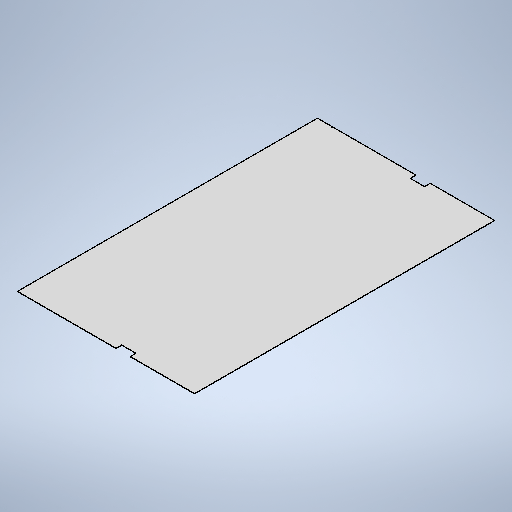
# Autodesk Inventor part: GnG frame 1.1 floor sheet 2
Saved by Autodesk Inventor 2025.3 (Build 293356000, 356)
## iProperties
Created: 2025-10-28
Part Number: GnG frame 1.1 floor sheet 2
Material: Stainless Steel
Document SubType Name: Sheet Metal
Designer: admin
Mass: 280.619 g
Surface Area: 364.406 cm^2
Volume: 35.0774 cm^3
Density: 8 g/cm^3
Sheet Metal Rule: AISI304 3mm Die 32
Sheet Metal Width: 1240,000 mm
Sheet Metal Length: 2100,000 mm
Sheet Metal Area: 2604000,000 mm^2
Appearance: Default
Stock Number: 1.2
Flat Pattern Width: 124 cm
Flat Pattern Length: 210 cm
Flat Pattern Area: 26040 cm^2
Author: admin
Autodesk Inventor part; units mm, degrees
ref_plane "YZ Plane" through (0, 0, 0) normal (1, 0, 0) x (0, 1, 0)
ref_plane "XZ Plane" through (0, 0, 0) normal (0, 1, 0) x (-1, 0, 0)
ref_plane "XY Plane" through (0, 0, 0) normal (0, 0, 1) x (1, 0, 0)
sketch "Sketch1" plane through (0, 0, 0) normal (0, 0, 1) x (1, 0, 0)
  line L0 (0, 0) -> (-1240, 0)
  line L1 (-1240, 0) -> (-1240, -2100)
  line L2 (-1240, -2100) -> (0, -2100)
  line L3 (0, -2100) -> (0, 0)
  line L4 (0, 0) -> (-40, 0)
  line L5 (-40, 0) -> (-40, -40)
  line L6 (-40, -40) -> (0, -40)
  line L7 (0, -40) -> (0, 0)
  line L8 (0, -2100) -> (-40, -2100)
  line L9 (-40, -2100) -> (-40, -2060)
  line L10 (-40, -2060) -> (0, -2060)
  line L11 (0, -2060) -> (0, -2100)
  line L12 (-1240, 0) -> (-1200, 0)
  line L13 (-1200, 0) -> (-1200, -40)
  line L14 (-1200, -40) -> (-1240, -40)
  line L15 (-1240, -40) -> (-1240, 0)
  line L16 (-1240, -2100) -> (-1200, -2100)
  line L17 (-1200, -2100) -> (-1200, -2060)
  line L18 (-1200, -2060) -> (-1240, -2060)
  line L19 (-1240, -2060) -> (-1240, -2100)
  line L20 (-550, -2100) -> (-450, -2100)
  line L21 (-450, -2100) -> (-450, -2060)
  line L22 (-450, -2060) -> (-550, -2060)
  line L23 (-550, -2060) -> (-550, -2100)
  line L24 (-550, 0) -> (-450, 0)
  line L25 (-450, 0) -> (-450, -40)
  line L26 (-450, -40) -> (-550, -40)
  line L27 (-550, -40) -> (-550, 0)
  point P0 (0, -40)
  point P1 (-40, 0)
  point P2 (-40, -2100)
  point P3 (0, -2060)
  point P4 (-450, -2100)
  point P5 (-450, 0)
  dimension "d22" = 1240
  dimension "d23" = 2100
  dimension "d24" = 40
  dimension "d25" = 40
  dimension "d28" = 100
  dimension "d29" = 410
  measures "d22" distance of L2.end L1.end
  measures "d23" distance of L1.end L0.end
  measures "d24" distance of L6.end L5.end
  measures "d25" distance of L5.end L4.end
  measures "d28" distance of L25.end L26.end
  measures "d29" distance between parallel lines of L5 L25
extrude "Plate1" add sketch "Sketch1" along normal blind 3 contours L3 L6 L5 L0 | L5 L6 L3 L10 L9 L2 L21 L22 L23 L17 L18 L1 L14 L13 L0 L27 L26 L25 | L3 L2 L9 L10 | L13 L14 L1 L0 | L18 L17 L2 L1
sketch "Sketch6" plane through (0, 0, 3) normal (0, 0, 1) x (1, 0, 0)
  line L0 (0, 0) -> (0, -2100) projected
  line L1 (-450, 0) -> (0, 0) projected
  line L2 (-450, -40) -> (-450, 0) projected
  line L3 (-550, -40) -> (-450, -40) projected
  line L4 (-550, 0) -> (-550, -40) projected
  line L5 (-1240, 0) -> (-550, 0) projected
  line L6 (-1240, -2100) -> (-1240, 0) projected
  line L7 (-550, -2100) -> (-1240, -2100) projected
  line L8 (-550, -2060) -> (-550, -2100) projected
  line L9 (-450, -2060) -> (-550, -2060) projected
  line L10 (-450, -2100) -> (-450, -2060) projected
  line L11 (0, -2100) -> (-450, -2100) projected
  line L12 (-1135, 0) -> (-1133, 0)
  line L13 (-1133, 0) -> (-1133, -5)
  line L14 (-1133, -5) -> (-1135, -5)
  line L15 (-1135, -5) -> (-1135, 0)
  line L16 (-1127, 0) -> (-1125, 0)
  line L17 (-1125, 0) -> (-1125, -5)
  line L18 (-1125, -5) -> (-1127, -5)
  line L19 (-1127, -5) -> (-1127, 0)
  line L20 (-1131, 0) -> (-1129, 0)
  line L21 (-1129, 0) -> (-1129, -5)
  line L22 (-1129, -5) -> (-1131, -5)
  line L23 (-1131, -5) -> (-1131, 0)
  line L24 (-1133, -2.5) -> (-1131, -2.5)
  line L25 (-1123, 0) -> (-1120, 0)
  line L26 (-1129, -2.5) -> (-1127, -2.5)
  line L27 (-1123, 0) -> (-1121.9884, -4.6072)
  arc A0 (-1121.9884, -4.6072) -> (-1121.0116, -4.6072) centre (-1121.5, -4.5) ccw
  line L28 (-1121.0116, -4.6072) -> (-1120, 0)
  line L29 (-1125, 0) -> (-1123, 0)
  line L30 (-1112, -5) -> (-1114, -5)
  line L31 (-1112, -2.5) -> (-1110, -2.5)
  line L32 (-1116, -5) -> (-1118, -5)
  line L33 (-1116, -2.5) -> (-1114, -2.5)
  line L34 (-1114, 0) -> (-1112, 0)
  line L35 (-1114, -5) -> (-1114, 0)
  line L36 (-1118, 0) -> (-1116, 0)
  line L37 (-1118, -5) -> (-1118, 0)
  line L38 (-1116, 0) -> (-1116, -5)
  line L39 (-1112, 0) -> (-1112, -5)
  line L40 (-1110, -5) -> (-1110, 0)
  line L41 (-1110, 0) -> (-1108, 0)
  line L42 (-1108, 0) -> (-1108, -5)
  line L43 (-1108, -5) -> (-1110, -5)
  line L44 (-1120, 0) -> (-1118, 0)
  circle A1 centre (-1140, 0) radius 1.5
  line L45 (-1240, 0) -> (-550, 0) projected
  point P0 (-1121.5, 0)
  point P1 (-1138.5, 0)
  point P2 (-1141.5, 0)
  point P3 (-1133, 0)
  point P4 (-1135, 0)
  point P5 (-1129, 0)
  point P6 (-1131, 0)
  dimension "d38" = 2
  dimension "d39" = 5
  dimension "d40" = 0.5
  dimension "d41" = 3
  dimension "d42" = 2
  dimension "d43" = 5
  dimension "d44" = 3
  dimension "d45" = 5
  dimension "d46" = 100
  constraints: 66 end point, 12 parallel, 11 horizontal, 10 equal length, 9 midpoint, 6 perpendicular, 5 collinear, 3 tangent, 2 centre point, 2 point on circle, 2 point on line, 1 vertical alignment
  measures "d38" distance of L13.end L14.end
  measures "d39" distance of L14.end L12.start
  measures "d40" radius of A0
  measures "d41" distance of L29.end L25.end
  measures "d42" distance of L32.start L37.start
  measures "d43" distance of L37.start L44.end
  measures "d44" diameter of A1
  measures "d45" distance of A1.centre L12.start
  measures "d46" distance from line of L6 A1.centre
extrude "Cut1" cut sketch "Sketch6" against normal blind 3 contours L5 A1 | L5 L13 L14 L15 | L5 L21 L22 L23 picked at (-1140.0603, -0.4964)
equation "\"d24\" = d25"
equation "\"d40\" = 0.25 * d38"
equation "\"d47\" = Thickness"
equation "\"d2\" = Thickness"
equation "\"BendReliefWidth\" = Thickness"
equation "\"BendReliefDepth\" = 0.5 * Thickness"
equation "\"CornerReliefSize\" = 4 * Thickness"
equation "\"MinimumRemnant\" = 2 * Thickness"
equation "\"TransitionRadius\" = BendRadius"
equation "\"JacobiRadiusSize\" = BendRadius"
equation "\"GapSize\" = Thickness"
equation "\"Thickness\" = 3"
equation "\"BendRadius\" = 5"
body "Solid1"
